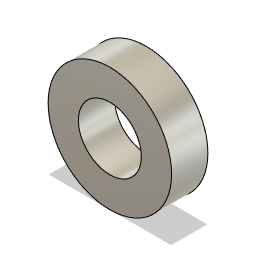
_Aluminum spacer m5.18793d64-0a1d-4db6-916d-4da26e1ae961 (Autodesk Fusion 360 design; units mm, degrees)
Autodesk Fusion 360 part; units mm, degrees
sketch "Sketch1" plane through (0, 0, 0) normal (0, 0, 1) x (1, 0, 0)
  circle A0 centre (0, 0) radius 2.6
  circle A1 centre (0, 0) radius 5.1
  dimension "d1" = 5.2
  dimension "d2" = 2.5
  constraint coincident A0.centre A1.centre
  measures "d1" diameter of A0
extrude "Extrude1" add sketch "Sketch1" along normal blind 3 makes body 1
extrude "Extrude2" add sketch "Sketch1" along normal blind 6 separate body makes body 2
copy_body "Body->Comp1" bodies 1 removing the originals makes body 3 in component "3MM SPACER"
copy_body "Body->Comp2" bodies 2 removing the originals makes body 4 in component "6MM SPACER"
component "3MM SPACER" placed x (1, 0, 0) y (0, 1, 0) z (0, 0, 1) at (0, 0, 0)
component "6MM SPACER" placed x (1, 0, 0) y (0, 1, 0) z (0, 0, 1) at (0, 0, 0)
named bodies: "3MM SPACER", "6MM SPACER"
